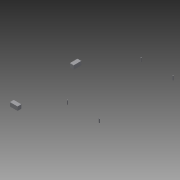
# Autodesk Inventor part: Wheelbase
Saved by Autodesk Inventor 2015 (Build 190159000, 159)
## iProperties
Created: 2016-01-19
Part Number: Wheelbase
Material: Generic
Document SubType Name: Modeling
Designer: sethbattis
Density: 1 g/cm^3
Appearance: Default
Author: sethbattis
Autodesk Inventor part; units mm, degrees
ref_plane "YZ Plane" through (0, 0, 0) normal (1, 0, 0) x (0, 1, 0)
ref_plane "XZ Plane" through (0, 0, 0) normal (0, 1, 0) x (-1, 0, 0)
ref_plane "XY Plane" through (0, 0, 0) normal (0, 0, 1) x (1, 0, 0)
sketch "Sketch1" plane through (0, 0, 0) normal (0, 1, 0) x (-1, 0, 0)
  line L0 (430.53, 0) -> (-405.13, 0) construction
  line L1 (0, -600.71) -> (0, 626.11) construction
  line L2 (285.75, 425.45) -> (-285.75, 425.45) construction
  line L3 (-285.75, 425.45) -> (-285.75, -425.45) construction
  line L4 (-285.75, -425.45) -> (285.75, -425.45) construction
  line L5 (285.75, -425.45) -> (285.75, 425.45) construction
  circle A0 centre (106.0958, 245.7958) radius 179.6542 construction
  circle A1 centre (106.0958, -245.7958) radius 179.6542 construction
  circle A2 centre (-106.0958, 245.7958) radius 179.6542 construction
  circle A3 centre (-106.0958, -245.7958) radius 179.6542 construction
  line L6 (106.0958, 245.7958) -> (106.0958, -245.7958) construction
  line L7 (-106.0958, 245.7958) -> (-106.0958, -245.7958) construction
  circle A4 centre (106.0958, 245.7958) radius 2.7781
  circle A5 centre (106.0958, -245.7958) radius 2.7781
  circle A6 centre (-106.0958, -245.7958) radius 2.7781
  circle A7 centre (-106.0958, 245.7958) radius 2.7781
  line L8 (311.15, -25.4) -> (285.75, -25.4)
  line L9 (285.75, -25.4) -> (285.75, 25.4)
  line L10 (285.75, 25.4) -> (311.15, 25.4)
  line L11 (311.15, 25.4) -> (311.15, -25.4)
  line L12 (285.75, 425.45) -> (234.95, 425.45)
  line L13 (234.95, 425.45) -> (234.95, 450.85)
  line L14 (234.95, 450.85) -> (285.75, 450.85)
  line L15 (285.75, 450.85) -> (285.75, 425.45)
  point P0 (0, 0)
  dimension "d2" = 850.9
  dimension "d3" = 571.5
  dimension "d8" = 359.3084
  dimension "d21" = 5.5563
  dimension "d24" = 25.4
  dimension "d25" = 50.8
  dimension "d26" = 50.8
  dimension "d27" = 25.4
  constraints: 28 end point, 8 centre point, 8 tangent, 6 equal radius, 6 parallel, 4 coincident, 3 horizontal, 3 perpendicular, 2 vertical, 1 collinear, 3 other
  measures "d2" distance of L4.end L2.start
  measures "d3" distance of L2.start L2.end
  measures "d8" diameter of A0
  measures "d21" diameter of A4
  measures "d24" distance of L9.end L10.end
  measures "d25" distance of L8.end L9.end
  measures "d26" distance of L13.end L14.end
  measures "d27" distance of L12.end L13.end
extrude "Extrusion3" add sketch "Sketch1" along normal blind 25.4
body "Solid3"
